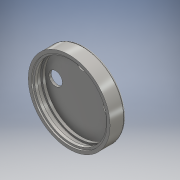
# Autodesk Inventor part: UR5 Palm
Saved by Autodesk Inventor 2016 (Build 200138000, 138)
## iProperties
Created: 2017-12-25
Part Number: UR5 Palm
Material: Aluminum 6061-AHC
Document SubType Name: Modeling
Designer: kornbot
Density: 2.7 g/cm^3
Appearance: Aluminum - Dark
Author: kornbot
Autodesk Inventor part; units mm, degrees
ref_plane "YZ Plane" through (0, 0, 0) normal (1, 0, 0) x (0, 1, 0)
ref_plane "XZ Plane" through (0, 0, 0) normal (0, 1, 0) x (-1, 0, 0)
ref_plane "XY Plane" through (0, 0, 0) normal (0, 0, 1) x (1, 0, 0)
sketch "Sketch1" plane through (0, 0, 0) normal (0, 0, 1) x (1, 0, 0)
  line L0 (0, 0) -> (0, 14)
  line L1 (0, 14) -> (-39.1825, 14)
  line L2 (-39.1825, 14) -> (-39, 0)
  line L3 (-39.1825, 14) -> (-42.1825, 14)
  line L4 (-42.1825, 14) -> (-39, 14)
  line L5 (-39, 14) -> (-39, 0)
  line L6 (-39, 0) -> (-42.1825, 0)
  line L7 (-42.1825, 0) -> (-42.1825, 14)
  line L8 (-39, 0) -> (-39, 5)
  line L9 (-39, 5) -> (-39, 9)
  line L10 (-39, 5) -> (-39, 4.5)
  line L11 (-39, 4.5) -> (-39, 1.5)
  line L12 (-39, 9) -> (-39, 9.5)
  line L13 (-39, 9.5) -> (-39, 12.5)
  line L14 (-39.1631, 12.5112) -> (-37.1631, 12.5112)
  line L15 (-39, 4.5) -> (-37, 4.5)
  line L16 (-37.1631, 12.5112) -> (-39, 12.5112)
  line L17 (-39, 12.5112) -> (-39, 9.5)
  line L18 (-39, 9.5) -> (-37.1631, 9.5)
  line L19 (-37.1631, 9.5) -> (-37.1631, 12.5112)
  line L20 (-37, 4.5) -> (-39, 4.5)
  line L21 (-39, 4.5) -> (-39, 1.5)
  line L22 (-39, 1.5) -> (-37, 1.5)
  line L23 (-37, 1.5) -> (-37, 4.5)
  dimension "d0" = 14
  dimension "d2" = 39.1825
  dimension "d3" = 3
  dimension "d4" = 5
  dimension "d5" = 4
  dimension "d6" = 0.5
  dimension "d7" = 3
  dimension "d8" = 0.5
  dimension "d9" = 3
  dimension "d10" = 2
  dimension "d11" = 2
  constraints: 48 end point, 7 horizontal, 7 point on line, 6 parallel, 3 perpendicular, 1 vertical
  measures "d0" distance of L0.start L0.end
  measures "d2" distance of L0.end L1.end
  measures "d3" distance of L1.end L3.end
  measures "d4" distance of L2.end L8.end
  measures "d5" distance of L8.end L9.end
  measures "d6" distance of L8.end L10.end
  measures "d7" distance of L10.end L11.end
  measures "d8" distance of L9.end L12.end
  measures "d9" distance of L12.end L13.end
  measures "d10" distance of L14.start L14.end
  measures "d11" distance of L10.end L15.end
revolve "Revolution1" add sketch "Sketch1" angle 360 about axis through (0, 0, 0) along (0, 1, 0) contours L2 L6 L7 L3 | L14 L19 L18 L5 | L5 L15 L23 L22
sketch "Sketch2" plane through (0, 14, 0) normal (0, 1, 0) x (1, 0, 0)
  circle A0 centre (0, 0) radius 42.0476
  constraints: 1 centre point, 1 coincident
extrude "Extrusion1" add sketch "Sketch2" along normal blind 2.5
sketch "Sketch3" plane through (0, 16.5, 0) normal (0, 1, 0) x (1, 0, 0)
  line L0 (0, 0) -> (0, -39)
  circle A0 centre (0, 0) radius 39 projected
  line L1 (0, 0) -> (10, 0)
  line L2 (0, 0) -> (-10, 0)
  line L3 (10, 0) -> (10, 33)
  line L4 (5, 0) -> (5, -8)
  line L5 (-5, 0) -> (-5, -8)
  line L6 (10, 0) -> (-12, 0)
  line L7 (-12, 0) -> (-12, 37.108)
  line L8 (-12, 37.108) -> (10, 37.108)
  line L9 (10, 37.108) -> (10, 0)
  line L10 (5, 0) -> (10, 0)
  line L11 (-5, 0) -> (-12, 0)
  line L12 (8, 0) -> (8, -8)
  line L13 (-8.5, 0) -> (-8.5, -8)
  line L14 (8, -8) -> (-9, -8)
  line L15 (-9, -8) -> (-9, -16.8367)
  line L16 (-9, -16.8367) -> (8, -16.8367)
  line L17 (8, -16.8367) -> (8, -8)
  dimension "d15" = 10
  dimension "d16" = 10
  constraints: 36 end point, 6 vertical, 4 parallel, 3 horizontal, 3 midpoint, 3 perpendicular, 2 point on circle, 2 point on line, 1 collinear
  measures "d15" distance of L1.start L1.end
  measures "d16" distance of L1.start L2.end
extrude "Extrusion2" add sketch "Sketch3" along normal blind 20 contours L2 L6 L7 L8 L9 L3 L1 | L14 L17 L16 L0 | L0 L16 L15 L14
sketch "Sketch4" plane through (0, 36.5, 0) normal (0, 1, 0) x (1, 0, 0)
  line L0 (-9, -8) -> (8, -8) projected
  line L1 (-9, -16.8367) -> (-9, -8) projected
  line L2 (8, -8) -> (-9, -8)
  line L3 (-9, -8) -> (-9, -16.8367)
  line L4 (-9, -16.8367) -> (8, -16.8367)
  line L5 (8, -16.8367) -> (8, -8)
  point P0 (0, 0)
  constraints: 8 end point, 2 parallel, 1 horizontal, 1 perpendicular
extrude "Extrusion3" cut sketch "Sketch4" against normal blind 5.25
sketch "Sketch5" plane through (-12, 16.5, -37.108) normal (-1, 0, 0) x (0, 0, 1)
  line L0 (37.108, 20) -> (45.5585, 14.75)
  line L1 (45.5585, 14.75) -> (45.5585, 0)
  line L2 (37.108, 0) -> (0, 0) projected
  line L3 (45.5585, 0) -> (37.108, 0)
  line L4 (37.108, 0) -> (37.108, 20)
  point P0 (37.108, -16.5)
  constraints: 8 end point, 1 collinear, 1 perpendicular, 1 vertical
extrude "Extrusion4" add sketch "Sketch5" against normal blind 22
fillet "Fillet1" radius 2 1 edges at (-42.0476, 16.5, 0)
sketch "Sketch6" plane through (0, 16.5, 0) normal (0, 1, 0) x (1, 0, 0)
  circle A0 centre (0, 0) radius 40.0476 projected
  line L0 (-12, 37.108) -> (10, 37.108) projected
  line L1 (9.1, 39) -> (-10, 39)
  line L2 (-10, 39) -> (-10, 37.108)
  line L3 (-10, 37.108) -> (9.1, 37.108)
  line L4 (9.1, 37.108) -> (9.1, 39)
  line L5 (9.1, 39) -> (-10, 39)
  line L6 (-10, 39) -> (-10, 36.6014)
  line L7 (-10, 36.6014) -> (9.1, 36.6014)
  line L8 (9.1, 36.6014) -> (9.1, 39)
  constraints: 16 end point, 4 parallel, 2 horizontal, 2 perpendicular, 1 point on line, 2 other
extrude "Extrusion5" add sketch "Sketch6" along normal blind 18.75 contours L4 L0 L2 A0 L1 | L2 L1 A0
sketch "Sketch7" plane through (-9.1, 16.5, -39) normal (0, 0, -1) x (-1, 0, 0)
  line L0 (0.9, 0) -> (0.9, 18.75) projected
  line L1 (0.9, 18.75) -> (-18, 18.75)
  line L2 (-18, 18.75) -> (-18, 0)
  line L3 (-18, 0) -> (0.9, 0)
  line L4 (0.9, 0) -> (0.9, 18.75)
  point P0 (-9.1, -16.5)
  constraints: 8 end point, 2 parallel, 1 horizontal, 1 perpendicular
extrude "Extrusion6" add sketch "Sketch7" along normal blind 1.25
fillet "Fillet2" radius 3 1 edges at (-0.55, 35.25, -40.25)
fillet "Fillet3" radius 0.75 1 edges at (-1, 36.5, -37.108)
sketch "Sketch8" plane through (-12, 16.5, 8.4505) normal (-1, 0, 0) x (0, 0, 1)
  arc A0 (-44.8085, 20) -> (-45.5585, 19.25) centre (-44.8085, 19.25) ccw projected
  line L0 (-45.5585, 0) -> (-45.5585, 19.25) projected
  line L1 (-44.8085, 20) -> (-35.8085, 20)
  line L2 (-8.4505, 20) -> (-44.8085, 20) projected
  line L3 (-35.8085, 20) -> (-35.8085, 27)
  line L4 (-44.8085, 20) -> (-35.8085, 27)
  point P0 (-8.4505, -16.5)
  dimension "d32" = 9
  dimension "d33" = 7
  constraints: 6 end point, 1 point on line, 1 vertical
  measures "d32" distance of L1.start L1.end
  measures "d33" distance of L1.end L3.end
extrude "Extrusion7" add sketch "Sketch8" against normal blind 22
fillet "Fillet4" radius 0.5 1 edges at (-1, 43.5, -27.358)
sketch "Sketch9" plane through (-12, 36.5, -36.358) normal (0, 0.7894, -0.6139) x (1, 0, 0)
  line L0 (21.9896, 0) -> (0, 0)
  line L1 (0, 0) -> (0, -11)
  line L2 (0, -11) -> (21.9896, -11)
  line L3 (21.9896, -11) -> (21.9896, 0)
  line L4 (0, 0) -> (22, 0) projected
  line L5 (0, -23.0909) -> (0, 12.8708) projected
  line L6 (0, -5.5) -> (21.9896, -0.3552)
  line L7 (21.9896, -5.5) -> (0, 0)
  circle A0 centre (19.2617, -2.8418) radius 1.5
  circle A1 centre (3.4617, -2.8418) radius 1.5
  point P0 (12, -6.2904)
  dimension "d41" = 3
  dimension "d42" = 3
  constraints: 12 end point, 2 centre point, 2 parallel, 2 point on line, 1 horizontal, 1 midpoint, 1 perpendicular
  measures "d41" diameter of A0
  measures "d42" diameter of A1
extrude "Extrusion8" cut sketch "Sketch9" against normal blind 22 contours A0 | A1
sketch "Sketch10" plane through (0, 16.5, 0) normal (0, 1, 0) x (1, 0, 0)
  circle A0 centre (0.1244, -27.7846) radius 7
  circle A1 centre (0, 0) radius 40.0476
  circle A2 centre (24, 14) radius 7
  circle A3 centre (-24.1244, 13.7846) radius 7
  circle A4 centre (28, 0) radius 7
  circle A5 centre (-28, 0) radius 7
  dimension "d45" = 14
  dimension "d48" = 360
  dimension "d50" = 14
  dimension "d51" = 14
  constraints: 6 centre point, 1 coincident, 7 other
  measures "d45" diameter of A0
  measures "d50" diameter of A4
  measures "d51" diameter of A5
extrude "Extrusion9" cut sketch "Sketch10" against normal blind 22 contours A0 | A4 | A5
fillet "Fillet5" radius 11.5 1 edges at (-1, 36.5, 0)
sketch "Sketch11" plane through (0, 36.5, 0) normal (0, 1, 0) x (1, 0, 0)
  line L0 (10, 27.358) -> (-12, 27.358) projected
  line L1 (-12, -8.4505) -> (-12, 37.108) projected
  circle A0 centre (-1, 15.3197) radius 8
  point P0 (0, 0)
  point P1 (10, 3.2814)
  point P2 (-12, 3.2814)
  dimension "d56" = 16
  constraints: 1 centre point
  measures "d56" diameter of A0
extrude "Extrusion10" cut sketch "Sketch11" against normal blind 7.5
body "Solid1"
